Autodesk Fusion 360 part; units mm, degrees
note: some values were not read from the file. Set by a fixed rule: which sketch regions a step uses.
(part 2 of 4)
  point P212 (95, 17.5)
  point P213 (115, 17.5)
  point P214 (135, 17.5)
  point P215 (155, 17.5)
  point P216 (175, 17.5)
  point P217 (195, 17.5)
  point P218 (115, 27.5)
  point P219 (135, 27.5)
  point P220 (155, 27.5)
  point P221 (175, 27.5)
  point P222 (115, 37.5)
  point P223 (135, 37.5)
  point P224 (155, 37.5)
  point P225 (175, 37.5)
  point P226 (-180, 12.5)
  dimension "d22" = 90
  dimension "d23" = 70
  dimension "d24" = 90
  dimension "d26" = 35
  dimension "d46" = 10
  dimension "d47" = 10
  dimension "d48" = 3
  dimension "d49" = 10
  dimension "d50" = 10
  dimension "d51" = 3
  dimension "d56" = 10
  dimension "d57" = 3
  dimension "d60" = 20
  dimension "d61" = 10
  dimension "d65" = 90
  dimension "d67" = 16
  dimension "d68" = 16
  constraint horizontal L9
  constraint parallel L9 L10
  constraint tangent L10 A0
  constraint horizontal L13
  constraint parallel L13 L14
  constraint tangent A4 L14
  constraint horizontal L17
  constraint parallel L17 L18
  constraint horizontal L460
  constraint midpoint L2 L460.start
  constraint symmetric L458.end L460 L462.start
  constraint horizontal L466
  constraint horizontal L467
  constraint horizontal L468
  measures "d22" distance of L5.start L5.end
  measures "d23" distance of L1.start L0.end
  measures "d24" horizontal distance of L1.start L1.end
  measures "d26" horizontal distance of L1.end L4.start
  measures "d46" distance of A1.centre A0.centre
  measures "d47" distance of L10.start L10.end
  measures "d48" distance of L9.end L10.start
  measures "d49" distance of A4.centre A5.centre
  measures "d50" distance of L14.end A4.end
  measures "d51" distance of A4.end L13.end
  measures "d56" distance of L18.start L18.end
  measures "d57" distance of L17.end L18.start
  measures "d65" distance of L457.end L458.end
  measures "d67" vertical distance of A6.centre A215.centre
  measures "d68" vertical distance of A5.centre A215.centre
extrude "Extrude1" add sketch "Sketch2" along normal blind 5
fillet "Fillet1" radius 10 4 edges at (360, 2.5, 107.5) (360, 2.5, 37.5) (-10, 2.5, 117.5) (-10, 2.5, 27.5)
fillet "Fillet3" radius 25 8 edges at (55, 2.5, 145) (55, 2.5, 0) (235, 2.5, 0) (235, 2.5, 145) (190, 2.5, 190) (100, 2.5, 190) (100, 2.5, -45) (190, 2.5, -45)
fillet "Fillet4" radius 15 4 edges at (215, 2.5, 145) (75, 2.5, 145) (215, 2.5, 0) (75, 2.5, 0)
sketch "Sketch4" plane through (0, 5, 0) normal (0, 1, 0) x (-1, 0, 0)
  arc A0 (-197.1438, -32.1411) -> (-175.2899, -45) centre (-175.2899, -20) ccw
  line L0 (-175.2899, -45) -> (-114.7101, -45)
  arc A1 (-114.7101, -45) -> (-92.8562, -32.1411) centre (-114.7101, -20) ccw
  line L1 (-92.8562, -32.1411) -> (-79.2863, -7.7154)
  arc A2 (-66.1739, 0) -> (-79.2863, -7.7154) centre (-66.1739, -15) ccw
  line L2 (-66.1739, 0) -> (-65.9975, 0)
  arc A3 (-65.9975, 0) -> (-47.5687, 8.1069) centre (-65.9975, 25) ccw
  line L3 (-47.5687, 8.1069) -> (-29.7917, 27.5)
  line L4 (-29.7917, 27.5) -> (0, 27.5)
  arc A4 (0, 27.5) -> (10, 37.5) centre (0, 37.5) ccw
  line L5 (10, 37.5) -> (10, 107.5)
  arc A5 (10, 107.5) -> (0, 117.5) centre (0, 107.5) ccw
  line L6 (0, 117.5) -> (-25, 117.5)
  line L7 (-25, 117.5) -> (-47.8315, 138.4289)
  arc A6 (-47.8315, 138.4289) -> (-64.7246, 145) centre (-64.7246, 120) ccw
  line L8 (-64.7246, 145) -> (-66.1739, 145)
  arc A7 (-79.2863, 152.7154) -> (-66.1739, 145) centre (-66.1739, 160) ccw
  line L9 (-79.2863, 152.7154) -> (-92.8562, 177.1411)
  arc A8 (-92.8562, 177.1411) -> (-114.7101, 190) centre (-114.7101, 165) ccw
  line L10 (-114.7101, 190) -> (-175.2899, 190)
  arc A9 (-175.2899, 190) -> (-197.1438, 177.1411) centre (-175.2899, 165) ccw
  line L11 (-197.1438, 177.1411) -> (-210.7137, 152.7154)
  arc A10 (-223.8261, 145) -> (-210.7137, 152.7154) centre (-223.8261, 160) ccw
  line L12 (-223.8261, 145) -> (-227.6575, 145)
  arc A11 (-227.6575, 145) -> (-241.1764, 141.0295) centre (-227.6575, 120) ccw
  line L13 (-241.1764, 141.0295) -> (-270, 122.5)
  line L14 (-270, 122.5) -> (-351.644, 108.8927)
  arc A12 (-351.644, 108.8927) -> (-360, 99.0287) centre (-350, 99.0287) ccw
  line L15 (-360, 99.0287) -> (-360, 45.9713)
  arc A13 (-360, 45.9713) -> (-351.644, 36.1073) centre (-350, 45.9713) ccw
  line L16 (-351.644, 36.1073) -> (-270, 22.5)
  line L17 (-270, 22.5) -> (-241.1764, 3.9705)
  arc A14 (-241.1764, 3.9705) -> (-227.6575, 0) centre (-227.6575, 25) ccw
  line L18 (-227.6575, 0) -> (-223.8261, 0)
  arc A15 (-210.7137, -7.7154) -> (-223.8261, 0) centre (-223.8261, -15) ccw
  line L19 (-210.7137, -7.7154) -> (-197.1438, -32.1411)
  arc A16 (-90, 141) -> (-90, 144) centre (-90, 142.5) ccw
  line L20 (-90, 141) -> (-100, 141)
  arc A17 (-100, 144) -> (-100, 141) centre (-100, 142.5) ccw
  line L21 (-100, 144) -> (-90, 144)
  arc A18 (-150, 141) -> (-150, 144) centre (-150, 142.5) ccw
  line L22 (-150, 141) -> (-160, 141)
  arc A19 (-160, 144) -> (-160, 141) centre (-160, 142.5) ccw
  line L23 (-160, 144) -> (-150, 144)
  arc A20 (-270, 101) -> (-270, 104) centre (-270, 102.5) ccw
  line L24 (-270, 101) -> (-280, 101)
  arc A21 (-280, 104) -> (-280, 101) centre (-280, 102.5) ccw
  line L25 (-280, 104) -> (-270, 104)
  arc A22 (-230, 101) -> (-230, 104) centre (-230, 102.5) ccw
  line L26 (-230, 101) -> (-240, 101)
  arc A23 (-240, 104) -> (-240, 101) centre (-240, 102.5) ccw
  line L27 (-240, 104) -> (-230, 104)
  arc A24 (-170, 141) -> (-170, 144) centre (-170, 142.5) ccw
  line L28 (-170, 141) -> (-180, 141)
  arc A25 (-180, 144) -> (-180, 141) centre (-180, 142.5) ccw
  line L29 (-180, 144) -> (-170, 144)
  arc A26 (-70, 131) -> (-70, 134) centre (-70, 132.5) ccw
  line L30 (-70, 131) -> (-80, 131)
  arc A27 (-80, 134) -> (-80, 131) centre (-80, 132.5) ccw
  line L31 (-80, 134) -> (-70, 134)
  arc A28 (-190, 101) -> (-190, 104) centre (-190, 102.5) ccw
  line L32 (-190, 101) -> (-200, 101)
  arc A29 (-200, 104) -> (-200, 101) centre (-200, 102.5) ccw
  line L33 (-200, 104) -> (-190, 104)
  arc A30 (-130, 171) -> (-130, 174) centre (-130, 172.5) ccw
  line L34 (-130, 171) -> (-140, 171)
  arc A31 (-140, 174) -> (-140, 171) centre (-140, 172.5) ccw
  line L35 (-140, 174) -> (-130, 174)
  arc A32 (-150, 171) -> (-150, 174) centre (-150, 172.5) ccw
  line L36 (-150, 171) -> (-160, 171)
  arc A33 (-160, 174) -> (-160, 171) centre (-160, 172.5) ccw
  line L37 (-160, 174) -> (-150, 174)
  arc A34 (-130, 161) -> (-130, 164) centre (-130, 162.5) ccw
  line L38 (-130, 161) -> (-140, 161)
  arc A35 (-140, 164) -> (-140, 161) centre (-140, 162.5) ccw
  line L39 (-140, 164) -> (-130, 164)
  arc A36 (-70, 91) -> (-70, 94) centre (-70, 92.5) ccw
  line L40 (-70, 91) -> (-80, 91)
  arc A37 (-80, 94) -> (-80, 91) centre (-80, 92.5) ccw
  line L41 (-80, 94) -> (-70, 94)
  arc A38 (-150, 111) -> (-150, 114) centre (-150, 112.5) ccw
  line L42 (-150, 111) -> (-160, 111)
  arc A39 (-160, 114) -> (-160, 111) centre (-160, 112.5) ccw
  line L43 (-160, 114) -> (-150, 114)
  arc A40 (-150, 161) -> (-150, 164) centre (-150, 162.5) ccw
  line L44 (-150, 161) -> (-160, 161)
  arc A41 (-160, 164) -> (-160, 161) centre (-160, 162.5) ccw
  line L45 (-160, 164) -> (-150, 164)
  arc A42 (-170, 131) -> (-170, 134) centre (-170, 132.5) ccw
  line L46 (-170, 131) -> (-180, 131)
  arc A43 (-180, 134) -> (-180, 131) centre (-180, 132.5) ccw
  line L47 (-180, 134) -> (-170, 134)
  arc A44 (-190, 141) -> (-190, 144) centre (-190, 142.5) ccw
  line L48 (-190, 141) -> (-200, 141)
  arc A45 (-200, 144) -> (-200, 141) centre (-200, 142.5) ccw
  line L49 (-200, 144) -> (-190, 144)
  arc A46 (-70, 111) -> (-70, 114) centre (-70, 112.5) ccw
  line L50 (-70, 111) -> (-80, 111)
  arc A47 (-80, 114) -> (-80, 111) centre (-80, 112.5) ccw
  line L51 (-80, 114) -> (-70, 114)
  arc A48 (-348.5, 58) -> (-348.5, 55) centre (-348.5, 56.5) ccw
  line L52 (-348.5, 58) -> (-338.5, 58)
  arc A49 (-338.5, 55) -> (-338.5, 58) centre (-338.5, 56.5) ccw
  line L53 (-338.5, 55) -> (-348.5, 55)
  arc A50 (-110, 131) -> (-110, 134) centre (-110, 132.5) ccw
  line L54 (-110, 131) -> (-120, 131)
  arc A51 (-120, 134) -> (-120, 131) centre (-120, 132.5) ccw
  line L55 (-120, 134) -> (-110, 134)
  arc A52 (-130, 151) -> (-130, 154) centre (-130, 152.5) ccw
  line L56 (-130, 151) -> (-140, 151)
  arc A53 (-140, 154) -> (-140, 151) centre (-140, 152.5) ccw
  line L57 (-140, 154) -> (-130, 154)
  arc A54 (-170, 111) -> (-170, 114) centre (-170, 112.5) ccw
  line L58 (-170, 111) -> (-180, 111)
  arc A55 (-180, 114) -> (-180, 111) centre (-180, 112.5) ccw
  line L59 (-180, 114) -> (-170, 114)
  arc A56 (-25, 90) -> (-25, 87) centre (-25, 88.5) ccw
  line L60 (-25, 90) -> (-15, 90)
  arc A57 (-15, 87) -> (-15, 90) centre (-15, 88.5) ccw
  line L61 (-15, 87) -> (-25, 87)
  arc A58 (-70, 101) -> (-70, 104) centre (-70, 102.5) ccw
  line L62 (-70, 101) -> (-80, 101)
  arc A59 (-80, 104) -> (-80, 101) centre (-80, 102.5) ccw
  line L63 (-80, 104) -> (-70, 104)
  arc A60 (-250, 101) -> (-250, 104) centre (-250, 102.5) ccw
  line L64 (-250, 101) -> (-260, 101)
  arc A61 (-260, 104) -> (-260, 101) centre (-260, 102.5) ccw
  line L65 (-260, 104) -> (-250, 104)
  arc A62 (-90, 101) -> (-90, 104) centre (-90, 102.5) ccw
  line L66 (-90, 101) -> (-100, 101)
  arc A63 (-100, 104) -> (-100, 101) centre (-100, 102.5) ccw
  line L67 (-100, 104) -> (-90, 104)
  arc A64 (-210, 131) -> (-210, 134) centre (-210, 132.5) ccw
  line L68 (-210, 131) -> (-220, 131)
  arc A65 (-220, 134) -> (-220, 131) centre (-220, 132.5) ccw
  line L69 (-220, 134) -> (-210, 134)
  arc A66 (-130, 101) -> (-130, 104) centre (-130, 102.5) ccw
  line L70 (-130, 101) -> (-140, 101)
  arc A67 (-140, 104) -> (-140, 101) centre (-140, 102.5) ccw
  line L71 (-140, 104) -> (-130, 104)
  arc A68 (-90, 131) -> (-90, 134) centre (-90, 132.5) ccw
  line L72 (-90, 131) -> (-100, 131)
  arc A69 (-100, 134) -> (-100, 131) centre (-100, 132.5) ccw
  line L73 (-100, 134) -> (-90, 134)
  arc A70 (-170, 171) -> (-170, 174) centre (-170, 172.5) ccw
  line L74 (-170, 171) -> (-180, 171)
  arc A71 (-180, 174) -> (-180, 171) centre (-180, 172.5) ccw
  line L75 (-180, 174) -> (-170, 174)
  arc A72 (-110, 171) -> (-110, 174) centre (-110, 172.5) ccw
  line L76 (-110, 171) -> (-120, 171)
  arc A73 (-120, 174) -> (-120, 171) centre (-120, 172.5) ccw
  line L77 (-120, 174) -> (-110, 174)
  arc A74 (-170, 101) -> (-170, 104) centre (-170, 102.5) ccw
  line L78 (-170, 101) -> (-180, 101)
  arc A75 (-180, 104) -> (-180, 101) centre (-180, 102.5) ccw
  line L79 (-180, 104) -> (-170, 104)
  arc A76 (-90, 161) -> (-90, 164) centre (-90, 162.5) ccw
  line L80 (-90, 161) -> (-100, 161)
  arc A77 (-100, 164) -> (-100, 161) centre (-100, 162.5) ccw
  line L81 (-100, 164) -> (-90, 164)
  arc A78 (-210, 121) -> (-210, 124) centre (-210, 122.5) ccw
  line L82 (-210, 121) -> (-220, 121)
  arc A79 (-220, 124) -> (-220, 121) centre (-220, 122.5) ccw
  line L83 (-220, 124) -> (-210, 124)
  arc A80 (-150, 151) -> (-150, 154) centre (-150, 152.5) ccw
  line L84 (-150, 151) -> (-160, 151)
  arc A81 (-160, 154) -> (-160, 151) centre (-160, 152.5) ccw
  line L85 (-160, 154) -> (-150, 154)
  arc A82 (-210, 111) -> (-210, 114) centre (-210, 112.5) ccw
  line L86 (-210, 111) -> (-220, 111)
  arc A83 (-220, 114) -> (-220, 111) centre (-220, 112.5) ccw
  line L87 (-220, 114) -> (-210, 114)
  arc A84 (-130, 141) -> (-130, 144) centre (-130, 142.5) ccw
  line L88 (-130, 141) -> (-140, 141)
  arc A85 (-140, 144) -> (-140, 141) centre (-140, 142.5) ccw
  line L89 (-140, 144) -> (-130, 144)
  arc A86 (-190, 91) -> (-190, 94) centre (-190, 92.5) ccw
  line L90 (-190, 91) -> (-200, 91)
  arc A87 (-200, 94) -> (-200, 91) centre (-200, 92.5) ccw
  line L91 (-200, 94) -> (-190, 94)
  arc A88 (-250, 111) -> (-250, 114) centre (-250, 112.5) ccw
  line L92 (-250, 111) -> (-260, 111)
  arc A89 (-260, 114) -> (-260, 111) centre (-260, 112.5) ccw
  line L93 (-260, 114) -> (-250, 114)
  arc A90 (-130, 121) -> (-130, 124) centre (-130, 122.5) ccw
  line L94 (-130, 121) -> (-140, 121)
  arc A91 (-140, 124) -> (-140, 121) centre (-140, 122.5) ccw
  line L95 (-140, 124) -> (-130, 124)
  arc A92 (-130, 181) -> (-130, 184) centre (-130, 182.5) ccw
  line L96 (-130, 181) -> (-140, 181)
  arc A93 (-140, 184) -> (-140, 181) centre (-140, 182.5) ccw
  line L97 (-140, 184) -> (-130, 184)
  arc A94 (-270, 111) -> (-270, 114) centre (-270, 112.5) ccw
  line L98 (-270, 111) -> (-280, 111)
  arc A95 (-280, 114) -> (-280, 111) centre (-280, 112.5) ccw
  line L99 (-280, 114) -> (-270, 114)
  arc A96 (-90, 111) -> (-90, 114) centre (-90, 112.5) ccw
  line L100 (-90, 111) -> (-100, 111)
  arc A97 (-100, 114) -> (-100, 111) centre (-100, 112.5) ccw
  line L101 (-100, 114) -> (-90, 114)
  arc A98 (-170, 181) -> (-170, 184) centre (-170, 182.5) ccw
  line L102 (-170, 181) -> (-180, 181)
  arc A99 (-180, 184) -> (-180, 181) centre (-180, 182.5) ccw
  line L103 (-180, 184) -> (-170, 184)
  arc A100 (-10, 101) -> (-10, 104) centre (-10, 102.5) ccw
  line L104 (-10, 101) -> (-20, 101)
  arc A101 (-20, 104) -> (-20, 101) centre (-20, 102.5) ccw
  line L105 (-20, 104) -> (-10, 104)
  arc A102 (-150, 181) -> (-150, 184) centre (-150, 182.5) ccw
  line L106 (-150, 181) -> (-160, 181)
  arc A103 (-160, 184) -> (-160, 181) centre (-160, 182.5) ccw
  line L107 (-160, 184) -> (-150, 184)
  arc A104 (-150, 131) -> (-150, 134) centre (-150, 132.5) ccw
  line L108 (-150, 131) -> (-160, 131)
  arc A105 (-160, 134) -> (-160, 131) centre (-160, 132.5) ccw
  line L109 (-160, 134) -> (-150, 134)
  arc A106 (-110, 181) -> (-110, 184) centre (-110, 182.5) ccw
  line L110 (-110, 181) -> (-120, 181)
  arc A107 (-120, 184) -> (-120, 181) centre (-120, 182.5) ccw
  line L111 (-120, 184) -> (-110, 184)
  arc A108 (-110, 161) -> (-110, 164) centre (-110, 162.5) ccw
  line L112 (-110, 161) -> (-120, 161)
  arc A109 (-120, 164) -> (-120, 161) centre (-120, 162.5) ccw
  line L113 (-120, 164) -> (-110, 164)
  arc A110 (-110, 91) -> (-110, 94) centre (-110, 92.5) ccw
  line L114 (-110, 91) -> (-120, 91)
  arc A111 (-120, 94) -> (-120, 91) centre (-120, 92.5) ccw
  line L115 (-120, 94) -> (-110, 94)
  arc A112 (-170, 91) -> (-170, 94) centre (-170, 92.5) ccw
  line L116 (-170, 91) -> (-180, 91)
  arc A113 (-180, 94) -> (-180, 91) centre (-180, 92.5) ccw
  line L117 (-180, 94) -> (-170, 94)
  arc A114 (-170, 121) -> (-170, 124) centre (-170, 122.5) ccw
  line L118 (-170, 121) -> (-180, 121)
  arc A115 (-180, 124) -> (-180, 121) centre (-180, 122.5) ccw
  line L119 (-180, 124) -> (-170, 124)
  arc A116 (-50, 101) -> (-50, 104) centre (-50, 102.5) ccw
  line L120 (-50, 101) -> (-60, 101)
  arc A117 (-60, 104) -> (-60, 101) centre (-60, 102.5) ccw
  line L121 (-60, 104) -> (-50, 104)
  arc A118 (-150, 101) -> (-150, 104) centre (-150, 102.5) ccw
  line L122 (-150, 101) -> (-160, 101)
  arc A119 (-160, 104) -> (-160, 101) centre (-160, 102.5) ccw
  line L123 (-160, 104) -> (-150, 104)
  arc A120 (-50, 111) -> (-50, 114) centre (-50, 112.5) ccw
  line L124 (-50, 111) -> (-60, 111)
  arc A121 (-60, 114) -> (-60, 111) centre (-60, 112.5) ccw
  line L125 (-60, 114) -> (-50, 114)
  arc A122 (-150, 91) -> (-150, 94) centre (-150, 92.5) ccw
  line L126 (-150, 91) -> (-160, 91)
  arc A123 (-160, 94) -> (-160, 91) centre (-160, 92.5) ccw
  line L127 (-160, 94) -> (-150, 94)
  arc A124 (-190, 111) -> (-190, 114) centre (-190, 112.5) ccw
  line L128 (-190, 111) -> (-200, 111)
  arc A125 (-200, 114) -> (-200, 111) centre (-200, 112.5) ccw
  line L129 (-200, 114) -> (-190, 114)
  arc A126 (-50, 81) -> (-50, 84) centre (-50, 82.5) ccw
  line L130 (-50, 81) -> (-60, 81)
  arc A127 (-60, 84) -> (-60, 81) centre (-60, 82.5) ccw
  line L131 (-60, 84) -> (-50, 84)
  arc A128 (-310, 91) -> (-310, 94) centre (-310, 92.5) ccw
  line L132 (-310, 91) -> (-320, 91)
  arc A129 (-320, 94) -> (-320, 91) centre (-320, 92.5) ccw
  line L133 (-320, 94) -> (-310, 94)
  arc A130 (-190, 81) -> (-190, 84) centre (-190, 82.5) ccw
  line L134 (-190, 81) -> (-200, 81)
  arc A131 (-200, 84) -> (-200, 81) centre (-200, 82.5) ccw
  line L135 (-200, 84) -> (-190, 84)
  arc A132 (-250, 81) -> (-250, 84) centre (-250, 82.5) ccw
  line L136 (-250, 81) -> (-260, 81)
  arc A133 (-260, 84) -> (-260, 81) centre (-260, 82.5) ccw
  line L137 (-260, 84) -> (-250, 84)
  arc A134 (-90, -19) -> (-90, -16) centre (-90, -17.5) ccw
  line L138 (-90, -19) -> (-100, -19)
  arc A135 (-100, -16) -> (-100, -19) centre (-100, -17.5) ccw
  line L139 (-100, -16) -> (-90, -16)
  arc A136 (-310, 81) -> (-310, 84) centre (-310, 82.5) ccw
  line L140 (-310, 81) -> (-320, 81)
  arc A137 (-320, 84) -> (-320, 81) centre (-320, 82.5) ccw
  line L141 (-320, 84) -> (-310, 84)
  arc A138 (-190, -9) -> (-190, -6) centre (-190, -7.5) ccw
  line L142 (-190, -9) -> (-200, -9)
  arc A139 (-200, -6) -> (-200, -9) centre (-200, -7.5) ccw
  line L143 (-200, -6) -> (-190, -6)
  arc A140 (-130, 81) -> (-130, 84) centre (-130, 82.5) ccw
  line L144 (-130, 81) -> (-140, 81)
  arc A141 (-140, 84) -> (-140, 81) centre (-140, 82.5) ccw
  line L145 (-140, 84) -> (-130, 84)
  arc A142 (-50, 71) -> (-50, 74) centre (-50, 72.5) ccw
  line L146 (-50, 71) -> (-60, 71)
  arc A143 (-60, 74) -> (-60, 71) centre (-60, 72.5) ccw
  line L147 (-60, 74) -> (-50, 74)
  arc A144 (-90, 81) -> (-90, 84) centre (-90, 82.5) ccw
  line L148 (-90, 81) -> (-100, 81)
  arc A145 (-100, 84) -> (-100, 81) centre (-100, 82.5) ccw
  line L149 (-100, 84) -> (-90, 84)
  arc A146 (-270, 91) -> (-270, 94) centre (-270, 92.5) ccw
  line L150 (-270, 91) -> (-280, 91)
  arc A147 (-280, 94) -> (-280, 91) centre (-280, 92.5) ccw
  line L151 (-280, 94) -> (-270, 94)
  arc A148 (-150, -19) -> (-150, -16) centre (-150, -17.5) ccw
  line L152 (-150, -19) -> (-160, -19)
  arc A149 (-160, -16) -> (-160, -19) centre (-160, -17.5) ccw
  line L153 (-160, -16) -> (-150, -16)
  arc A150 (-130, -19) -> (-130, -16) centre (-130, -17.5) ccw
  line L154 (-130, -19) -> (-140, -19)
  arc A151 (-140, -16) -> (-140, -19) centre (-140, -17.5) ccw
  line L155 (-140, -16) -> (-130, -16)
  arc A152 (-190, -19) -> (-190, -16) centre (-190, -17.5) ccw
  line L156 (-190, -19) -> (-200, -19)
  arc A153 (-200, -16) -> (-200, -19) centre (-200, -17.5) ccw
  line L157 (-200, -16) -> (-190, -16)
  arc A154 (-290, 91) -> (-290, 94) centre (-290, 92.5) ccw
  line L158 (-290, 91) -> (-300, 91)
  arc A155 (-300, 94) -> (-300, 91) centre (-300, 92.5) ccw
  line L159 (-300, 94) -> (-290, 94)
  arc A156 (-170, -19) -> (-170, -16) centre (-170, -17.5) ccw
  line L160 (-170, -19) -> (-180, -19)
  arc A157 (-180, -16) -> (-180, -19) centre (-180, -17.5) ccw
  line L161 (-180, -16) -> (-170, -16)
  arc A158 (-130, -29) -> (-130, -26) centre (-130, -27.5) ccw
  line L162 (-130, -29) -> (-140, -29)
  arc A159 (-140, -26) -> (-140, -29) centre (-140, -27.5) ccw
  line L163 (-140, -26) -> (-130, -26)
  arc A160 (-290, 81) -> (-290, 84) centre (-290, 82.5) ccw
  line L164 (-290, 81) -> (-300, 81)
  arc A161 (-300, 84) -> (-300, 81) centre (-300, 82.5) ccw
  line L165 (-300, 84) -> (-290, 84)
  arc A162 (-110, -29) -> (-110, -26) centre (-110, -27.5) ccw
  line L166 (-110, -29) -> (-120, -29)
  arc A163 (-120, -26) -> (-120, -29) centre (-120, -27.5) ccw
  line L167 (-120, -26) -> (-110, -26)
  arc A164 (-170, -29) -> (-170, -26) centre (-170, -27.5) ccw
  line L168 (-170, -29) -> (-180, -29)
  arc A165 (-180, -26) -> (-180, -29) centre (-180, -27.5) ccw
  line L169 (-180, -26) -> (-170, -26)
  arc A166 (-270, 81) -> (-270, 84) centre (-270, 82.5) ccw
  line L170 (-270, 81) -> (-280, 81)
  arc A167 (-280, 84) -> (-280, 81) centre (-280, 82.5) ccw
  line L171 (-280, 84) -> (-270, 84)
  arc A168 (-150, -29) -> (-150, -26) centre (-150, -27.5) ccw
  line L172 (-150, -29) -> (-160, -29)
  arc A169 (-160, -26) -> (-160, -29) centre (-160, -27.5) ccw
  line L173 (-160, -26) -> (-150, -26)
  arc A170 (-190, 71) -> (-190, 74) centre (-190, 72.5) ccw
  line L174 (-190, 71) -> (-200, 71)
  arc A171 (-200, 74) -> (-200, 71) centre (-200, 72.5) ccw
  line L175 (-200, 74) -> (-190, 74)
  arc A172 (-130, -39) -> (-130, -36) centre (-130, -37.5) ccw
  line L176 (-130, -39) -> (-140, -39)
  arc A173 (-140, -36) -> (-140, -39) centre (-140, -37.5) ccw
  line L177 (-140, -36) -> (-130, -36)
  arc A174 (-210, 71) -> (-210, 74) centre (-210, 72.5) ccw
  line L178 (-210, 71) -> (-220, 71)
  arc A175 (-220, 74) -> (-220, 71) centre (-220, 72.5) ccw
  line L179 (-220, 74) -> (-210, 74)
  arc A176 (-110, -39) -> (-110, -36) centre (-110, -37.5) ccw
  line L180 (-110, -39) -> (-120, -39)
  arc A177 (-120, -36) -> (-120, -39) centre (-120, -37.5) ccw
  line L181 (-120, -36) -> (-110, -36)
  arc A178 (-90, 71) -> (-90, 74) centre (-90, 72.5) ccw
  line L182 (-90, 71) -> (-100, 71)
  arc A179 (-100, 74) -> (-100, 71) centre (-100, 72.5) ccw
  line L183 (-100, 74) -> (-90, 74)
  arc A180 (-230, 71) -> (-230, 74) centre (-230, 72.5) ccw
  line L184 (-230, 71) -> (-240, 71)
  arc A181 (-240, 74) -> (-240, 71) centre (-240, 72.5) ccw
  line L185 (-240, 74) -> (-230, 74)
  arc A182 (-170, -39) -> (-170, -36) centre (-170, -37.5) ccw
  line L186 (-170, -39) -> (-180, -39)
  arc A183 (-180, -36) -> (-180, -39) centre (-180, -37.5) ccw
  line L187 (-180, -36) -> (-170, -36)
  arc A184 (-150, 71) -> (-150, 74) centre (-150, 72.5) ccw
  line L188 (-150, 71) -> (-160, 71)
  arc A185 (-160, 74) -> (-160, 71) centre (-160, 72.5) ccw
  line L189 (-160, 74) -> (-150, 74)
  arc A186 (-150, 81) -> (-150, 84) centre (-150, 82.5) ccw
  line L190 (-150, 81) -> (-160, 81)
  arc A187 (-160, 84) -> (-160, 81) centre (-160, 82.5) ccw
  line L191 (-160, 84) -> (-150, 84)
  arc A188 (-150, -39) -> (-150, -36) centre (-150, -37.5) ccw
  line L192 (-150, -39) -> (-160, -39)
  arc A189 (-160, -36) -> (-160, -39) centre (-160, -37.5) ccw
  line L193 (-160, -36) -> (-150, -36)
  arc A190 (-210, 81) -> (-210, 84) centre (-210, 82.5) ccw
  line L194 (-210, 81) -> (-220, 81)
  arc A191 (-220, 84) -> (-220, 81) centre (-220, 82.5) ccw
  line L195 (-220, 84) -> (-210, 84)
  arc A192 (-70, 71) -> (-70, 74) centre (-70, 72.5) ccw
  line L196 (-70, 71) -> (-80, 71)
  arc A193 (-80, 74) -> (-80, 71) centre (-80, 72.5) ccw
  line L197 (-80, 74) -> (-70, 74)
  arc A194 (-30, 71) -> (-30, 74) centre (-30, 72.5) ccw
  line L198 (-30, 71) -> (-40, 71)
  arc A195 (-40, 74) -> (-40, 71) centre (-40, 72.5) ccw
  line L199 (-40, 74) -> (-30, 74)
  arc A196 (-110, 81) -> (-110, 84) centre (-110, 82.5) ccw
  line L200 (-110, 81) -> (-120, 81)
  arc A197 (-120, 84) -> (-120, 81) centre (-120, 82.5) ccw
  line L201 (-120, 84) -> (-110, 84)
  arc A198 (-110, 71) -> (-110, 74) centre (-110, 72.5) ccw
  line L202 (-110, 71) -> (-120, 71)
  arc A199 (-120, 74) -> (-120, 71) centre (-120, 72.5) ccw
  line L203 (-120, 74) -> (-110, 74)
  arc A200 (-230, 81) -> (-230, 84) centre (-230, 82.5) ccw
  line L204 (-230, 81) -> (-240, 81)
  arc A201 (-240, 84) -> (-240, 81) centre (-240, 82.5) ccw
  line L205 (-240, 84) -> (-230, 84)
  arc A202 (-130, 71) -> (-130, 74) centre (-130, 72.5) ccw
  line L206 (-130, 71) -> (-140, 71)
  arc A203 (-140, 74) -> (-140, 71) centre (-140, 72.5) ccw
  line L207 (-140, 74) -> (-130, 74)
  arc A204 (-170, 81) -> (-170, 84) centre (-170, 82.5) ccw
  line L208 (-170, 81) -> (-180, 81)
  arc A205 (-180, 84) -> (-180, 81) centre (-180, 82.5) ccw
  line L209 (-180, 84) -> (-170, 84)
  arc A206 (-70, 81) -> (-70, 84) centre (-70, 82.5) ccw
  line L210 (-70, 81) -> (-80, 81)
  arc A207 (-80, 84) -> (-80, 81) centre (-80, 82.5) ccw
  line L211 (-80, 84) -> (-70, 84)
  arc A208 (-90, 151) -> (-90, 154) centre (-90, 152.5) ccw
  line L212 (-90, 151) -> (-100, 151)
  arc A209 (-100, 154) -> (-100, 151) centre (-100, 152.5) ccw
  line L213 (-100, 154) -> (-90, 154)
  arc A210 (-50, 131) -> (-50, 134) centre (-50, 132.5) ccw
  line L214 (-50, 131) -> (-60, 131)
  arc A211 (-60, 134) -> (-60, 131) centre (-60, 132.5) ccw
  line L215 (-60, 134) -> (-50, 134)
  arc A212 (-338.5, 87) -> (-338.5, 90) centre (-338.5, 88.5) ccw
  line L216 (-338.5, 87) -> (-348.5, 87)
  arc A213 (-348.5, 90) -> (-348.5, 87) centre (-348.5, 88.5) ccw
  line L217 (-348.5, 90) -> (-338.5, 90)
  arc A214 (-50, 121) -> (-50, 124) centre (-50, 122.5) ccw
  line L218 (-50, 121) -> (-60, 121)
  arc A215 (-60, 124) -> (-60, 121) centre (-60, 122.5) ccw
  line L219 (-60, 124) -> (-50, 124)
  arc A216 (-190, 161) -> (-190, 164) centre (-190, 162.5) ccw
  line L220 (-190, 161) -> (-200, 161)
  arc A217 (-200, 164) -> (-200, 161) centre (-200, 162.5) ccw
  line L221 (-200, 164) -> (-190, 164)
  arc A218 (-70, 121) -> (-70, 124) centre (-70, 122.5) ccw
  line L222 (-70, 121) -> (-80, 121)
  arc A219 (-80, 124) -> (-80, 121) centre (-80, 122.5) ccw
  line L223 (-80, 124) -> (-70, 124)
  arc A220 (-230, 121) -> (-230, 124) centre (-230, 122.5) ccw
  line L224 (-230, 121) -> (-240, 121)
  arc A221 (-240, 124) -> (-240, 121) centre (-240, 122.5) ccw
  line L225 (-240, 124) -> (-230, 124)
  arc A222 (-180, 74) -> (-180, 71) centre (-180, 72.5) ccw
  line L226 (-180, 74) -> (-170, 74)
  arc A223 (-170, 71) -> (-170, 74) centre (-170, 72.5) ccw
  line L227 (-170, 71) -> (-180, 71)
  arc A224 (-130, 91) -> (-130, 94) centre (-130, 92.5) ccw
  line L228 (-130, 91) -> (-140, 91)
  arc A225 (-140, 94) -> (-140, 91) centre (-140, 92.5) ccw
  line L229 (-140, 94) -> (-130, 94)
  arc A226 (-190, 131) -> (-190, 134) centre (-190, 132.5) ccw
  line L230 (-190, 131) -> (-200, 131)
  arc A227 (-200, 134) -> (-200, 131) centre (-200, 132.5) ccw
  line L231 (-200, 134) -> (-190, 134)
  arc A228 (-170, 161) -> (-170, 164) centre (-170, 162.5) ccw
  line L232 (-170, 161) -> (-180, 161)
  arc A229 (-180, 164) -> (-180, 161) centre (-180, 162.5) ccw
  line L233 (-180, 164) -> (-170, 164)
  arc A230 (-110, 151) -> (-110, 154) centre (-110, 152.5) ccw
  line L234 (-110, 151) -> (-120, 151)
  arc A231 (-120, 154) -> (-120, 151) centre (-120, 152.5) ccw
  line L235 (-120, 154) -> (-110, 154)
  arc A232 (-130, 111) -> (-130, 114) centre (-130, 112.5) ccw
  line L236 (-130, 111) -> (-140, 111)
  arc A233 (-140, 114) -> (-140, 111) centre (-140, 112.5) ccw
  line L237 (-140, 114) -> (-130, 114)
  arc A234 (-25, 58) -> (-25, 55) centre (-25, 56.5) ccw
  line L238 (-25, 58) -> (-15, 58)
  arc A235 (-15, 55) -> (-15, 58) centre (-15, 56.5) ccw
  line L239 (-15, 55) -> (-25, 55)
  arc A236 (-170, 151) -> (-170, 154) centre (-170, 152.5) ccw
  line L240 (-170, 151) -> (-180, 151)
  arc A237 (-180, 154) -> (-180, 151) centre (-180, 152.5) ccw
  line L241 (-180, 154) -> (-170, 154)
  arc A238 (-90, 121) -> (-90, 124) centre (-90, 122.5) ccw
  line L242 (-90, 121) -> (-100, 121)
  arc A239 (-100, 124) -> (-100, 121) centre (-100, 122.5) ccw
  line L243 (-100, 124) -> (-90, 124)
  arc A240 (-110, 101) -> (-110, 104) centre (-110, 102.5) ccw
  line L244 (-110, 101) -> (-120, 101)
  arc A241 (-120, 104) -> (-120, 101) centre (-120, 102.5) ccw
  line L245 (-120, 104) -> (-110, 104)
  arc A242 (-310, 101) -> (-310, 104) centre (-310, 102.5) ccw
  line L246 (-310, 101) -> (-320, 101)
  arc A243 (-320, 104) -> (-320, 101) centre (-320, 102.5) ccw
  line L247 (-320, 104) -> (-310, 104)
  arc A244 (-250, 121) -> (-250, 124) centre (-250, 122.5) ccw
  line L248 (-250, 121) -> (-260, 121)
  arc A245 (-260, 124) -> (-260, 121) centre (-260, 122.5) ccw
  line L249 (-260, 124) -> (-250, 124)
  arc A246 (-230, 111) -> (-230, 114) centre (-230, 112.5) ccw
  line L250 (-230, 111) -> (-240, 111)
  arc A247 (-240, 114) -> (-240, 111) centre (-240, 112.5) ccw
  line L251 (-240, 114) -> (-230, 114)
  arc A248 (-110, 111) -> (-110, 114) centre (-110, 112.5) ccw
  line L252 (-110, 111) -> (-120, 111)
  arc A249 (-120, 114) -> (-120, 111) centre (-120, 112.5) ccw
  line L253 (-120, 114) -> (-110, 114)
  arc A250 (-290, 101) -> (-290, 104) centre (-290, 102.5) ccw
  line L254 (-290, 101) -> (-300, 101)
  arc A251 (-300, 104) -> (-300, 101) centre (-300, 102.5) ccw
  line L255 (-300, 104) -> (-290, 104)
  arc A252 (-190, 151) -> (-190, 154) centre (-190, 152.5) ccw
  line L256 (-190, 151) -> (-200, 151)
  arc A253 (-200, 154) -> (-200, 151) centre (-200, 152.5) ccw
  line L257 (-200, 154) -> (-190, 154)
  arc A254 (-230, 131) -> (-230, 134) centre (-230, 132.5) ccw
  line L258 (-230, 131) -> (-240, 131)
  arc A255 (-240, 134) -> (-240, 131) centre (-240, 132.5) ccw
  line L259 (-240, 134) -> (-230, 134)
  arc A256 (-130, 131) -> (-130, 134) centre (-130, 132.5) ccw
  line L260 (-130, 131) -> (-140, 131)
  arc A257 (-140, 134) -> (-140, 131) centre (-140, 132.5) ccw
  line L261 (-140, 134) -> (-130, 134)
  arc A258 (-110, 121) -> (-110, 124) centre (-110, 122.5) ccw
  line L262 (-110, 121) -> (-120, 121)
  arc A259 (-120, 124) -> (-120, 121) centre (-120, 122.5) ccw
  line L263 (-120, 124) -> (-110, 124)
  arc A260 (-250, 91) -> (-250, 94) centre (-250, 92.5) ccw
  line L264 (-250, 91) -> (-260, 91)
  arc A261 (-260, 94) -> (-260, 91) centre (-260, 92.5) ccw
  line L265 (-260, 94) -> (-250, 94)
  arc A262 (-210, 101) -> (-210, 104) centre (-210, 102.5) ccw
  line L266 (-210, 101) -> (-220, 101)
  arc A263 (-220, 104) -> (-220, 101) centre (-220, 102.5) ccw
  line L267 (-220, 104) -> (-210, 104)
  arc A264 (-210, 91) -> (-210, 94) centre (-210, 92.5) ccw
  line L268 (-210, 91) -> (-220, 91)
  arc A265 (-220, 94) -> (-220, 91) centre (-220, 92.5) ccw
  line L269 (-220, 94) -> (-210, 94)
  arc A266 (-230, 91) -> (-230, 94) centre (-230, 92.5) ccw
  line L270 (-230, 91) -> (-240, 91)
  arc A267 (-240, 94) -> (-240, 91) centre (-240, 92.5) ccw
  line L271 (-240, 94) -> (-230, 94)
  arc A268 (-110, -19) -> (-110, -16) centre (-110, -17.5) ccw
  line L272 (-110, -19) -> (-120, -19)
  arc A269 (-120, -16) -> (-120, -19) centre (-120, -17.5) ccw
  line L273 (-120, -16) -> (-110, -16)
  arc A270 (-230, 41) -> (-230, 44) centre (-230, 42.5) ccw
  line L274 (-230, 41) -> (-240, 41)
  arc A271 (-240, 44) -> (-240, 41) centre (-240, 42.5) ccw
  line L275 (-240, 44) -> (-230, 44)
  arc A272 (-250, 41) -> (-250, 44) centre (-250, 42.5) ccw
  line L276 (-250, 41) -> (-260, 41)
  arc A273 (-260, 44) -> (-260, 41) centre (-260, 42.5) ccw
  line L277 (-260, 44) -> (-250, 44)
  arc A274 (-30, 41) -> (-30, 44) centre (-30, 42.5) ccw
  line L278 (-30, 41) -> (-40, 41)
  arc A275 (-40, 44) -> (-40, 41) centre (-40, 42.5) ccw
  line L279 (-40, 44) -> (-30, 44)
  arc A276 (-290, 41) -> (-290, 44) centre (-290, 42.5) ccw
  line L280 (-290, 41) -> (-300, 41)
  arc A277 (-300, 44) -> (-300, 41) centre (-300, 42.5) ccw
  line L281 (-300, 44) -> (-290, 44)
  arc A278 (-190, 41) -> (-190, 44) centre (-190, 42.5) ccw
  line L282 (-190, 41) -> (-200, 41)
  arc A279 (-200, 44) -> (-200, 41) centre (-200, 42.5) ccw
  line L283 (-200, 44) -> (-190, 44)
  arc A280 (-70, 41) -> (-70, 44) centre (-70, 42.5) ccw
  line L284 (-70, 41) -> (-80, 41)
  arc A281 (-80, 44) -> (-80, 41) centre (-80, 42.5) ccw
  line L285 (-80, 44) -> (-70, 44)
  arc A282 (-50, 21) -> (-50, 24) centre (-50, 22.5) ccw
  line L286 (-50, 21) -> (-60, 21)
  arc A283 (-60, 24) -> (-60, 21) centre (-60, 22.5) ccw
  line L287 (-60, 24) -> (-50, 24)
  arc A284 (-110, 41) -> (-110, 44) centre (-110, 42.5) ccw
  line L288 (-110, 41) -> (-120, 41)
  arc A285 (-120, 44) -> (-120, 41) centre (-120, 42.5) ccw
  line L289 (-120, 44) -> (-110, 44)
  arc A286 (-150, 31) -> (-150, 34) centre (-150, 32.5) ccw
  line L290 (-150, 31) -> (-160, 31)
  arc A287 (-160, 34) -> (-160, 31) centre (-160, 32.5) ccw
  line L291 (-160, 34) -> (-150, 34)
  arc A288 (-90, 21) -> (-90, 24) centre (-90, 22.5) ccw
  line L292 (-90, 21) -> (-100, 21)
  arc A289 (-100, 24) -> (-100, 21) centre (-100, 22.5) ccw
  line L293 (-100, 24) -> (-90, 24)
  arc A290 (-70, 31) -> (-70, 34) centre (-70, 32.5) ccw
  line L294 (-70, 31) -> (-80, 31)
  arc A291 (-80, 34) -> (-80, 31) centre (-80, 32.5) ccw
  line L295 (-80, 34) -> (-70, 34)
  arc A292 (-170, 21) -> (-170, 24) centre (-170, 22.5) ccw
  line L296 (-170, 21) -> (-180, 21)
  arc A293 (-180, 24) -> (-180, 21) centre (-180, 22.5) ccw
  line L297 (-180, 24) -> (-170, 24)
  arc A294 (-10, 41) -> (-10, 44) centre (-10, 42.5) ccw
  line L298 (-10, 41) -> (-20, 41)
  arc A295 (-20, 44) -> (-20, 41) centre (-20, 42.5) ccw
  line L299 (-20, 44) -> (-10, 44)
  arc A296 (-210, 31) -> (-210, 34) centre (-210, 32.5) ccw
  line L300 (-210, 31) -> (-220, 31)
  arc A297 (-220, 34) -> (-220, 31) centre (-220, 32.5) ccw
  line L301 (-220, 34) -> (-210, 34)
  arc A298 (-250, 31) -> (-250, 34) centre (-250, 32.5) ccw
  line L302 (-250, 31) -> (-260, 31)
  arc A299 (-260, 34) -> (-260, 31) centre (-260, 32.5) ccw
  line L303 (-260, 34) -> (-250, 34)
  arc A300 (-210, 41) -> (-210, 44) centre (-210, 42.5) ccw
  line L304 (-210, 41) -> (-220, 41)
  arc A301 (-220, 44) -> (-220, 41) centre (-220, 42.5) ccw
  line L305 (-220, 44) -> (-210, 44)
  arc A302 (-310, 41) -> (-310, 44) centre (-310, 42.5) ccw
  line L306 (-310, 41) -> (-320, 41)
  arc A303 (-320, 44) -> (-320, 41) centre (-320, 42.5) ccw
  line L307 (-320, 44) -> (-310, 44)
  arc A304 (-130, 21) -> (-130, 24) centre (-130, 22.5) ccw
  line L308 (-130, 21) -> (-140, 21)
  arc A305 (-140, 24) -> (-140, 21) centre (-140, 22.5) ccw
  line L309 (-140, 24) -> (-130, 24)
  arc A306 (-130, 41) -> (-130, 44) centre (-130, 42.5) ccw
  line L310 (-130, 41) -> (-140, 41)
  arc A307 (-140, 44) -> (-140, 41) centre (-140, 42.5) ccw
  line L311 (-140, 44) -> (-130, 44)
  arc A308 (-170, 41) -> (-170, 44) centre (-170, 42.5) ccw
  line L312 (-170, 41) -> (-180, 41)
  arc A309 (-180, 44) -> (-180, 41) centre (-180, 42.5) ccw
  line L313 (-180, 44) -> (-170, 44)
  arc A310 (-110, 31) -> (-110, 34) centre (-110, 32.5) ccw
  line L314 (-110, 31) -> (-120, 31)
  arc A311 (-120, 34) -> (-120, 31) centre (-120, 32.5) ccw
  line L315 (-120, 34) -> (-110, 34)
  arc A312 (-270, 41) -> (-270, 44) centre (-270, 42.5) ccw
  line L316 (-270, 41) -> (-280, 41)
  arc A313 (-280, 44) -> (-280, 41) centre (-280, 42.5) ccw
  line L317 (-280, 44) -> (-270, 44)
  arc A314 (-90, 41) -> (-90, 44) centre (-90, 42.5) ccw
  line L318 (-90, 41) -> (-100, 41)
  arc A315 (-100, 44) -> (-100, 41) centre (-100, 42.5) ccw
  line L319 (-100, 44) -> (-90, 44)
  arc A316 (-130, 31) -> (-130, 34) centre (-130, 32.5) ccw
  line L320 (-130, 31) -> (-140, 31)
  arc A317 (-140, 34) -> (-140, 31) centre (-140, 32.5) ccw
  line L321 (-140, 34) -> (-130, 34)
  arc A318 (-50, 41) -> (-50, 44) centre (-50, 42.5) ccw
  line L322 (-50, 41) -> (-60, 41)
  arc A319 (-60, 44) -> (-60, 41) centre (-60, 42.5) ccw
  line L323 (-60, 44) -> (-50, 44)
  arc A320 (-110, 21) -> (-110, 24) centre (-110, 22.5) ccw
  line L324 (-110, 21) -> (-120, 21)
  arc A321 (-120, 24) -> (-120, 21) centre (-120, 22.5) ccw
  line L325 (-120, 24) -> (-110, 24)
  arc A322 (-170, 31) -> (-170, 34) centre (-170, 32.5) ccw
  line L326 (-170, 31) -> (-180, 31)
  arc A323 (-180, 34) -> (-180, 31) centre (-180, 32.5) ccw
  line L327 (-180, 34) -> (-170, 34)
  arc A324 (-170, 1) -> (-170, 4) centre (-170, 2.5) ccw
  line L328 (-170, 1) -> (-180, 1)
  arc A325 (-180, 4) -> (-180, 1) centre (-180, 2.5) ccw
  line L329 (-180, 4) -> (-170, 4)
  arc A326 (-150, 41) -> (-150, 44) centre (-150, 42.5) ccw
  line L330 (-150, 41) -> (-160, 41)
  arc A327 (-160, 44) -> (-160, 41) centre (-160, 42.5) ccw
  line L331 (-160, 44) -> (-150, 44)
  arc A328 (-150, -9) -> (-150, -6) centre (-150, -7.5) ccw
  line L332 (-150, -9) -> (-160, -9)
  arc A329 (-160, -6) -> (-160, -9) centre (-160, -7.5) ccw
  line L333 (-160, -6) -> (-150, -6)
  arc A330 (-50, 11) -> (-50, 14) centre (-50, 12.5) ccw
  line L334 (-50, 11) -> (-60, 11)
  arc A331 (-60, 14) -> (-60, 11) centre (-60, 12.5) ccw
  line L335 (-60, 14) -> (-50, 14)
  arc A332 (-90, -9) -> (-90, -6) centre (-90, -7.5) ccw
  line L336 (-90, -9) -> (-100, -9)
  arc A333 (-100, -6) -> (-100, -9) centre (-100, -7.5) ccw
  line L337 (-100, -6) -> (-90, -6)
  arc A334 (-110, 11) -> (-110, 14) centre (-110, 12.5) ccw
  line L338 (-110, 11) -> (-120, 11)
  arc A335 (-120, 14) -> (-120, 11) centre (-120, 12.5) ccw
  line L339 (-120, 14) -> (-110, 14)
  arc A336 (-170, -9) -> (-170, -6) centre (-170, -7.5) ccw
  line L340 (-170, -9) -> (-180, -9)
  arc A337 (-180, -6) -> (-180, -9) centre (-180, -7.5) ccw
  line L341 (-180, -6) -> (-170, -6)
  arc A338 (-150, 1) -> (-150, 4) centre (-150, 2.5) ccw
  line L342 (-150, 1) -> (-160, 1)
  arc A339 (-160, 4) -> (-160, 1) centre (-160, 2.5) ccw
  line L343 (-160, 4) -> (-150, 4)
  arc A340 (-190, 1) -> (-190, 4) centre (-190, 2.5) ccw
  line L344 (-190, 1) -> (-200, 1)
  arc A341 (-200, 4) -> (-200, 1) centre (-200, 2.5) ccw
  line L345 (-200, 4) -> (-190, 4)
  arc A342 (-130, -9) -> (-130, -6) centre (-130, -7.5) ccw
  line L346 (-130, -9) -> (-140, -9)
  arc A343 (-140, -6) -> (-140, -9) centre (-140, -7.5) ccw
  line L347 (-140, -6) -> (-130, -6)
  arc A344 (-130, 1) -> (-130, 4) centre (-130, 2.5) ccw
  line L348 (-130, 1) -> (-140, 1)
  arc A345 (-140, 4) -> (-140, 1) centre (-140, 2.5) ccw
  line L349 (-140, 4) -> (-130, 4)
  arc A346 (-230, 21) -> (-230, 24) centre (-230, 22.5) ccw
  line L350 (-230, 21) -> (-240, 21)
  arc A347 (-240, 24) -> (-240, 21) centre (-240, 22.5) ccw
  line L351 (-240, 24) -> (-230, 24)
  arc A348 (-110, 1) -> (-110, 4) centre (-110, 2.5) ccw
  line L352 (-110, 1) -> (-120, 1)
  arc A349 (-120, 4) -> (-120, 1) centre (-120, 2.5) ccw
  line L353 (-120, 4) -> (-110, 4)
  arc A350 (-150, 11) -> (-150, 14) centre (-150, 12.5) ccw
  line L354 (-150, 11) -> (-160, 11)
  arc A351 (-160, 14) -> (-160, 11) centre (-160, 12.5) ccw
  line L355 (-160, 14) -> (-150, 14)
  arc A352 (-170, 11) -> (-170, 14) centre (-170, 12.5) ccw
  line L356 (-170, 11) -> (-180, 11)
  arc A353 (-180, 14) -> (-180, 11) centre (-180, 12.5) ccw
  line L357 (-180, 14) -> (-170, 14)
  arc A354 (-210, 11) -> (-210, 14) centre (-210, 12.5) ccw
  line L358 (-210, 11) -> (-220, 11)
  arc A355 (-220, 14) -> (-220, 11) centre (-220, 12.5) ccw
  line L359 (-220, 14) -> (-210, 14)
  arc A356 (-230, 11) -> (-230, 14) centre (-230, 12.5) ccw
  line L360 (-230, 11) -> (-240, 11)
  arc A357 (-240, 14) -> (-240, 11) centre (-240, 12.5) ccw
  line L361 (-240, 14) -> (-230, 14)
  arc A358 (-70, 11) -> (-70, 14) centre (-70, 12.5) ccw
  line L362 (-70, 11) -> (-80, 11)
  arc A359 (-80, 14) -> (-80, 11) centre (-80, 12.5) ccw
  line L363 (-80, 14) -> (-70, 14)
  arc A360 (-90, 11) -> (-90, 14) centre (-90, 12.5) ccw
  line L364 (-90, 11) -> (-100, 11)
  arc A361 (-100, 14) -> (-100, 11) centre (-100, 12.5) ccw
  line L365 (-100, 14) -> (-90, 14)
  arc A362 (-250, 21) -> (-250, 24) centre (-250, 22.5) ccw
  line L366 (-250, 21) -> (-260, 21)
  arc A363 (-260, 24) -> (-260, 21) centre (-260, 22.5) ccw
  line L367 (-260, 24) -> (-250, 24)
  arc A364 (-130, 11) -> (-130, 14) centre (-130, 12.5) ccw
  line L368 (-130, 11) -> (-140, 11)
  arc A365 (-140, 14) -> (-140, 11) centre (-140, 12.5) ccw
  line L369 (-140, 14) -> (-130, 14)
  arc A366 (-190, 11) -> (-190, 14) centre (-190, 12.5) ccw
  line L370 (-190, 11) -> (-200, 11)
  arc A367 (-200, 14) -> (-200, 11) centre (-200, 12.5) ccw
  line L371 (-200, 14) -> (-190, 14)
  arc A368 (-90, 1) -> (-90, 4) centre (-90, 2.5) ccw
  line L372 (-90, 1) -> (-100, 1)
  arc A369 (-100, 4) -> (-100, 1) centre (-100, 2.5) ccw
  line L373 (-100, 4) -> (-90, 4)
  arc A370 (-290, 71) -> (-290, 74) centre (-290, 72.5) ccw
  line L374 (-290, 71) -> (-300, 71)
  arc A371 (-300, 74) -> (-300, 71) centre (-300, 72.5) ccw
  line L375 (-300, 74) -> (-290, 74)
  arc A372 (-70, 51) -> (-70, 54) centre (-70, 52.5) ccw
  line L376 (-70, 51) -> (-80, 51)
  arc A373 (-80, 54) -> (-80, 51) centre (-80, 52.5) ccw
  line L377 (-80, 54) -> (-70, 54)
  arc A374 (-110, 61) -> (-110, 64) centre (-110, 62.5) ccw
  line L378 (-110, 61) -> (-120, 61)
  arc A375 (-120, 64) -> (-120, 61) centre (-120, 62.5) ccw
  line L379 (-120, 64) -> (-110, 64)
  arc A376 (-190, 51) -> (-190, 54) centre (-190, 52.5) ccw
  line L380 (-190, 51) -> (-200, 51)
  arc A377 (-200, 54) -> (-200, 51) centre (-200, 52.5) ccw
  line L381 (-200, 54) -> (-190, 54)
  arc A378 (-190, 61) -> (-190, 64) centre (-190, 62.5) ccw
  line L382 (-190, 61) -> (-200, 61)
  arc A379 (-200, 64) -> (-200, 61) centre (-200, 62.5) ccw
  line L383 (-200, 64) -> (-190, 64)
  arc A380 (-270, 71) -> (-270, 74) centre (-270, 72.5) ccw
  line L384 (-270, 71) -> (-280, 71)
  arc A381 (-280, 74) -> (-280, 71) centre (-280, 72.5) ccw
  line L385 (-280, 74) -> (-270, 74)
  arc A382 (-150, 61) -> (-150, 64) centre (-150, 62.5) ccw
  line L386 (-150, 61) -> (-160, 61)
  arc A383 (-160, 64) -> (-160, 61) centre (-160, 62.5) ccw
  line L387 (-160, 64) -> (-150, 64)
  arc A384 (-70, 21) -> (-70, 24) centre (-70, 22.5) ccw
  line L388 (-70, 21) -> (-80, 21)
  arc A385 (-80, 24) -> (-80, 21) centre (-80, 22.5) ccw
  line L389 (-80, 24) -> (-70, 24)
  arc A386 (-190, 21) -> (-190, 24) centre (-190, 22.5) ccw
  line L390 (-190, 21) -> (-200, 21)
  arc A387 (-200, 24) -> (-200, 21) centre (-200, 22.5) ccw
  line L391 (-200, 24) -> (-190, 24)
  arc A388 (-210, 21) -> (-210, 24) centre (-210, 22.5) ccw
  line L392 (-210, 21) -> (-220, 21)
  arc A389 (-220, 24) -> (-220, 21) centre (-220, 22.5) ccw
  line L393 (-220, 24) -> (-210, 24)
  arc A390 (-310, 71) -> (-310, 74) centre (-310, 72.5) ccw
  line L394 (-310, 71) -> (-320, 71)
  arc A391 (-320, 74) -> (-320, 71) centre (-320, 72.5) ccw
  line L395 (-320, 74) -> (-310, 74)
  arc A392 (-210, 51) -> (-210, 54) centre (-210, 52.5) ccw
  line L396 (-210, 51) -> (-220, 51)
  arc A393 (-220, 54) -> (-220, 51) centre (-220, 52.5) ccw
  line L397 (-220, 54) -> (-210, 54)
  arc A394 (-190, 31) -> (-190, 34) centre (-190, 32.5) ccw
  line L398 (-190, 31) -> (-200, 31)
  arc A395 (-200, 34) -> (-200, 31) centre (-200, 32.5) ccw
  line L399 (-200, 34) -> (-190, 34)
  arc A396 (-150, 21) -> (-150, 24) centre (-150, 22.5) ccw
  line L400 (-150, 21) -> (-160, 21)
  arc A397 (-160, 24) -> (-160, 21) centre (-160, 22.5) ccw
  line L401 (-160, 24) -> (-150, 24)
  arc A398 (-50, 31) -> (-50, 34) centre (-50, 32.5) ccw
  line L402 (-50, 31) -> (-60, 31)
  arc A399 (-60, 34) -> (-60, 31) centre (-60, 32.5) ccw
  line L403 (-60, 34) -> (-50, 34)
  arc A400 (-90, 31) -> (-90, 34) centre (-90, 32.5) ccw
  line L404 (-90, 31) -> (-100, 31)
  arc A401 (-100, 34) -> (-100, 31) centre (-100, 32.5) ccw
  line L405 (-100, 34) -> (-90, 34)
  arc A402 (-210, 61) -> (-210, 64) centre (-210, 62.5) ccw
  line L406 (-210, 61) -> (-220, 61)
  arc A403 (-220, 64) -> (-220, 61) centre (-220, 62.5) ccw
  line L407 (-220, 64) -> (-210, 64)
  arc A404 (-150, 51) -> (-150, 54) centre (-150, 52.5) ccw
  line L408 (-150, 51) -> (-160, 51)
  arc A405 (-160, 54) -> (-160, 51) centre (-160, 52.5) ccw
  line L409 (-160, 54) -> (-150, 54)
  arc A406 (-270, 31) -> (-270, 34) centre (-270, 32.5) ccw
  line L410 (-270, 31) -> (-280, 31)
  arc A407 (-280, 34) -> (-280, 31) centre (-280, 32.5) ccw
  line L411 (-280, 34) -> (-270, 34)
  arc A408 (-130, 51) -> (-130, 54) centre (-130, 52.5) ccw
  line L412 (-130, 51) -> (-140, 51)
  arc A409 (-140, 54) -> (-140, 51) centre (-140, 52.5) ccw
  line L413 (-140, 54) -> (-130, 54)
  arc A410 (-230, 51) -> (-230, 54) centre (-230, 52.5) ccw
  line L414 (-230, 51) -> (-240, 51)
  arc A411 (-240, 54) -> (-240, 51) centre (-240, 52.5) ccw
  line L415 (-240, 54) -> (-230, 54)
  arc A412 (-230, 31) -> (-230, 34) centre (-230, 32.5) ccw
  line L416 (-230, 31) -> (-240, 31)
  arc A413 (-240, 34) -> (-240, 31) centre (-240, 32.5) ccw
  line L417 (-240, 34) -> (-230, 34)
  arc A414 (-290, 61) -> (-290, 64) centre (-290, 62.5) ccw
  line L418 (-290, 61) -> (-300, 61)
  arc A415 (-300, 64) -> (-300, 61) centre (-300, 62.5) ccw
  line L419 (-300, 64) -> (-290, 64)
  arc A416 (-170, 51) -> (-170, 54) centre (-170, 52.5) ccw
  line L420 (-170, 51) -> (-180, 51)
  arc A417 (-180, 54) -> (-180, 51) centre (-180, 52.5) ccw
  line L421 (-180, 54) -> (-170, 54)
  arc A418 (-250, 61) -> (-250, 64) centre (-250, 62.5) ccw
  line L422 (-250, 61) -> (-260, 61)
  arc A419 (-260, 64) -> (-260, 61) centre (-260, 62.5) ccw
  line L423 (-260, 64) -> (-250, 64)
  arc A420 (-310, 61) -> (-310, 64) centre (-310, 62.5) ccw
  line L424 (-310, 61) -> (-320, 61)
  arc A421 (-320, 64) -> (-320, 61) centre (-320, 62.5) ccw
  line L425 (-320, 64) -> (-310, 64)
  arc A422 (-50, 61) -> (-50, 64) centre (-50, 62.5) ccw
  line L426 (-50, 61) -> (-60, 61)
  arc A423 (-60, 64) -> (-60, 61) centre (-60, 62.5) ccw
  line L427 (-60, 64) -> (-50, 64)
  arc A424 (-110, -9) -> (-110, -6) centre (-110, -7.5) ccw
  line L428 (-110, -9) -> (-120, -9)
  arc A425 (-120, -6) -> (-120, -9) centre (-120, -7.5) ccw
  line L429 (-120, -6) -> (-110, -6)
  arc A426 (-90, 51) -> (-90, 54) centre (-90, 52.5) ccw
  line L430 (-90, 51) -> (-100, 51)
  arc A427 (-100, 54) -> (-100, 51) centre (-100, 52.5) ccw
  line L431 (-100, 54) -> (-90, 54)
  arc A428 (-90, 61) -> (-90, 64) centre (-90, 62.5) ccw
  line L432 (-90, 61) -> (-100, 61)
  arc A429 (-100, 64) -> (-100, 61) centre (-100, 62.5) ccw
  line L433 (-100, 64) -> (-90, 64)
  arc A430 (-250, 71) -> (-250, 74) centre (-250, 72.5) ccw
  line L434 (-250, 71) -> (-260, 71)
  arc A431 (-260, 74) -> (-260, 71) centre (-260, 72.5) ccw
  line L435 (-260, 74) -> (-250, 74)
  arc A432 (-170, 61) -> (-170, 64) centre (-170, 62.5) ccw
  line L436 (-170, 61) -> (-180, 61)
  arc A433 (-180, 64) -> (-180, 61) centre (-180, 62.5) ccw
  line L437 (-180, 64) -> (-170, 64)
  arc A434 (-250, 51) -> (-250, 54) centre (-250, 52.5) ccw
  line L438 (-250, 51) -> (-260, 51)
  arc A435 (-260, 54) -> (-260, 51) centre (-260, 52.5) ccw
  line L439 (-260, 54) -> (-250, 54)
  arc A436 (-130, 61) -> (-130, 64) centre (-130, 62.5) ccw
  line L440 (-130, 61) -> (-140, 61)
  arc A437 (-140, 64) -> (-140, 61) centre (-140, 62.5) ccw
  line L441 (-140, 64) -> (-130, 64)
  arc A438 (-230, 61) -> (-230, 64) centre (-230, 62.5) ccw
  line L442 (-230, 61) -> (-240, 61)
  arc A439 (-240, 64) -> (-240, 61) centre (-240, 62.5) ccw
  line L443 (-240, 64) -> (-230, 64)
  arc A440 (-70, 61) -> (-70, 64) centre (-70, 62.5) ccw
  line L444 (-70, 61) -> (-80, 61)
  arc A441 (-80, 64) -> (-80, 61) centre (-80, 62.5) ccw
  line L445 (-80, 64) -> (-70, 64)
  arc A442 (-270, 61) -> (-270, 64) centre (-270, 62.5) ccw
  line L446 (-270, 61) -> (-280, 61)
  arc A443 (-280, 64) -> (-280, 61) centre (-280, 62.5) ccw
  line L447 (-280, 64) -> (-270, 64)
  arc A444 (-270, 51) -> (-270, 54) centre (-270, 52.5) ccw
  line L448 (-270, 51) -> (-280, 51)
  arc A445 (-280, 54) -> (-280, 51) centre (-280, 52.5) ccw
  line L449 (-280, 54) -> (-270, 54)
  arc A446 (-110, 51) -> (-110, 54) centre (-110, 52.5) ccw
  line L450 (-110, 51) -> (-120, 51)
  arc A447 (-120, 54) -> (-120, 51) centre (-120, 52.5) ccw
  line L451 (-120, 54) -> (-110, 54)
  arc A448 (-50, 51) -> (-50, 54) centre (-50, 52.5) ccw
  line L452 (-50, 51) -> (-60, 51)
  arc A449 (-60, 54) -> (-60, 51) centre (-60, 52.5) ccw
  line L453 (-60, 54) -> (-50, 54)
  arc A450 (-290, 51) -> (-290, 54) centre (-290, 52.5) ccw
  line L454 (-290, 51) -> (-300, 51)
  arc A451 (-300, 54) -> (-300, 51) centre (-300, 52.5) ccw
  line L455 (-300, 54) -> (-290, 54)
  arc A452 (-310, 51) -> (-310, 54) centre (-310, 52.5) ccw
  line L456 (-310, 51) -> (-320, 51)
  arc A453 (-320, 54) -> (-320, 51) centre (-320, 52.5) ccw
  line L457 (-320, 54) -> (-310, 54)
  arc A454 (-190, 121) -> (-190, 124) centre (-190, 122.5) ccw
  line L458 (-190, 121) -> (-200, 121)
  arc A455 (-200, 124) -> (-200, 121) centre (-200, 122.5) ccw
  line L459 (-200, 124) -> (-190, 124)
  arc A456 (-150, 121) -> (-150, 124) centre (-150, 122.5) ccw
  line L460 (-150, 121) -> (-160, 121)
  arc A457 (-160, 124) -> (-160, 121) centre (-160, 122.5) ccw
  line L461 (-160, 124) -> (-150, 124)
  arc A458 (-110, 141) -> (-110, 144) centre (-110, 142.5) ccw
  line L462 (-110, 141) -> (-120, 141)
  arc A459 (-120, 144) -> (-120, 141) centre (-120, 142.5) ccw
  line L463 (-120, 144) -> (-110, 144)
  arc A460 (-90, 91) -> (-90, 94) centre (-90, 92.5) ccw
  line L464 (-90, 91) -> (-100, 91)
  arc A461 (-100, 94) -> (-100, 91) centre (-100, 92.5) ccw
  line L465 (-100, 94) -> (-90, 94)
  arc A462 (-50, 91) -> (-50, 94) centre (-50, 92.5) ccw
  line L466 (-50, 91) -> (-60, 91)
  arc A463 (-60, 94) -> (-60, 91) centre (-60, 92.5) ccw
  line L467 (-60, 94) -> (-50, 94)